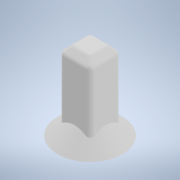
# Autodesk Inventor part: wheel_shtift
Saved by Autodesk Inventor 2022 (Build 260153000, 153)
## iProperties
Created: 2024-10-13
Part Number: wheel_shtift
Material: Типовые
Document SubType Name: Modeling
Designer: Andrey
Density: 1 g/cm^3
Appearance: По умолчанию
Author: Andrey
Autodesk Inventor part; units mm, degrees
ref_plane "YZ Plane" through (0, 0, 0) normal (1, 0, 0) x (0, 1, 0)
ref_plane "XZ Plane" through (0, 0, 0) normal (0, 1, 0) x (-1, 0, 0)
ref_plane "XY Plane" through (0, 0, 0) normal (0, 0, 1) x (1, 0, 0)
sketch "Эскиз1" plane through (0, 0, 0) normal (0, 1, 0) x (-1, 0, 0)
  circle A0 centre (0, 0) radius 4.95
  dimension "d0" = 9.9
  constraints: 1 centre point, 1 coincident
  measures "d0" diameter of A0
extrude "Выдавливание1" add sketch "Эскиз1" along normal blind 4.95
chamfer "Фаска1" distance 4.95 angle 45 1 edges at (4.95, 4.95, 0)
sketch "Эскиз2" plane through (0, 0, 0) normal (0, -1, 0) x (1, 0, 0)
  line L0 (-2.375, 2.375) -> (2.375, 2.375)
  line L1 (2.375, 2.375) -> (2.375, -2.375)
  line L2 (2.375, -2.375) -> (-2.375, -2.375)
  line L3 (-2.375, -2.375) -> (-2.375, 2.375)
  line L4 (-2.375, 2.375) -> (2.375, -2.375) construction
  line L5 (2.375, 2.375) -> (-2.375, -2.375) construction
  point P0 (0, 0)
  dimension "d6" = 4.75
  dimension "d7" = 4.75
  constraints: 12 end point, 2 midpoint, 2 parallel, 1 horizontal, 1 perpendicular
  measures "d6" distance of L1.end L2.end
  measures "d7" distance of L0.end L1.end
extrude "Выдавливание2" add sketch "Эскиз2" against normal blind 12
chamfer "Фаска2" distance 1 angle 45 4 edges at (0, 12, 2.375) (-2.375, 12, 0) (2.375, 12, 0) (0, 12, -2.375)
fillet "Сопряжение1" radius 0.7 16 edges at (-2.375, 6.2959, 2.375) (-1.875, 11.5, 1.875) (-1.875, 11.5, -1.875) (-2.375, 11, 0) (0, 11, -2.375) (0, 12, -1.375) (1.875, 11.5, -1.875) (2.375, 11, 0) (1.375, 12, 0) (-1.375, 12, 0) (1.875, 11.5, 1.875) (0, 11, 2.375) (0, 12, 1.375) (2.375, 6.2959, 2.375) (-2.375, 6.2959, -2.375) (2.375, 6.2959, -2.375)
